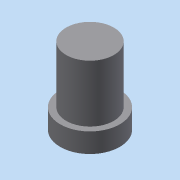
# Autodesk Inventor part: 00_IR_Laserdiode
Saved by Autodesk Inventor 2019.4 (Build 234330000, 330)
## iProperties
Created: 2020-11-30
Part Number: 00_IR_Laserdiode
Material: Generic
Document SubType Name: Modeling
Designer: diederichbenedict
Density: 1 g/cm^3
Appearance: Chrome - Polished
Author: diederichbenedict
Autodesk Inventor part; units mm, degrees
ref_plane "YZ Plane" through (0, 0, 0) normal (1, 0, 0) x (0, 1, 0)
ref_plane "XZ Plane" through (0, 0, 0) normal (0, 1, 0) x (-1, 0, 0)
ref_plane "XY Plane" through (0, 0, 0) normal (0, 0, 1) x (1, 0, 0)
sketch "Sketch1" plane through (0, 0, 0) normal (1, 0, 0) x (0, 1, 0)
  line L0 (0, 0) -> (9, 0)
  line L1 (9, 0) -> (9, -2.8)
  line L2 (9, -2.8) -> (2.3, -2.8)
  line L3 (2.3, -2.8) -> (2.3, -3.5)
  line L4 (2.3, -3.5) -> (0, -3.5)
  line L5 (0, -3.5) -> (0, 0)
  line L6 (0, -1.9829) -> (-0.9134, -1.9829)
  line L7 (-0.9134, -1.9829) -> (-0.9134, 0)
  line L8 (-0.9134, 0) -> (0, 0)
  dimension "d0" = 9
  dimension "d1" = 2.8
  dimension "d2" = 6.7
  dimension "d3" = 0.7
  constraints: 18 end point, 7 perpendicular, 2 horizontal, 2 point on line
  measures "d0" distance of L0.start L0.end
  measures "d1" distance of L0.end L1.end
  measures "d2" distance of L1.end L2.end
  measures "d3" distance of L2.end L3.end
revolve "Revolution1" add sketch "Sketch1" angle 360 about axis through (0, 0, 0) along (0, 1, 0)
body "Solid1"
